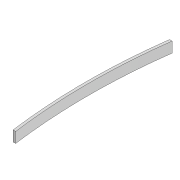
# Autodesk Inventor part: Support_strip
Saved by Autodesk Inventor 2022 (Build 260153000, 153)
## iProperties
Created: 2022-07-27
Part Number: Support_strip
Material: Generic
Document SubType Name: Modeling
Designer: dell
Density: 1 g/cm^3
Appearance: Default
Author: dell
Autodesk Inventor part; units mm, degrees
ref_plane "YZ Plane" through (0, 0, 0) normal (1, 0, 0) x (0, 1, 0)
ref_plane "XZ Plane" through (0, 0, 0) normal (0, 1, 0) x (-1, 0, 0)
ref_plane "XY Plane" through (0, 0, 0) normal (0, 0, 1) x (1, 0, 0)
sketch "Sketch1" plane through (0, 0, 0) normal (0, 1, 0) x (-1, 0, 0)
  arc A0 (0, -30) -> (0, 0) centre (-112, -15) ccw
  line L0 (0, 0) -> (0, -30) construction
  line L1 (0, -30) -> (1, -30) construction
  line L2 (1, -30) -> (1, 0) construction
  line L3 (1, 0) -> (0, 0) construction
  line L4 (0, 0) -> (0.5, 0)
  line L5 (0, -30) -> (0.5, -30)
  arc A1 (0.5, -30) -> (0.5, 0) centre (-111.7511, -15) ccw
  dimension "d0" = 30
  dimension "d1" = 1
  constraints: 12 end point, 4 point on circle, 2 centre point, 2 midpoint, 2 parallel, 2 tangent, 1 perpendicular, 1 vertical
  measures "d0" distance of L0.start L0.end
  measures "d1" distance of L1.end L0.end
extrude "Extrusion1" add sketch "Sketch1" along normal blind 2
body "Solid1"
